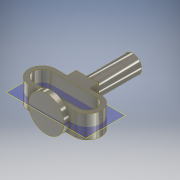
# Autodesk Inventor part: 부품1
Saved by Autodesk Inventor 2018 (Build 220112000, 112)
## iProperties
Created: 2019-05-21
Part Number: 부품1
Material: 은
Document SubType Name: Modeling
Designer: LeeYounSeo
Mass: 3715.59 g
Surface Area: 594.159 cm^2
Volume: 354.204 cm^3
Density: 10.49 g/cm^3
Appearance: 은
Author: LeeYounSeo
Autodesk Inventor part; units mm, degrees
ref_plane "YZ Plane" through (0, 0, 0) normal (1, 0, 0) x (0, 1, 0)
ref_plane "XZ Plane" through (0, 0, 0) normal (0, 1, 0) x (-1, 0, 0)
ref_plane "XY Plane" through (0, 0, 0) normal (0, 0, 1) x (1, 0, 0)
sketch "스케치1" plane through (0, 0, 0) normal (0, 0, 1) x (1, 0, 0)
  line L0 (-50, -20) -> (50, -20)
  line L1 (50, 20) -> (-50, 20)
  line L2 (-50, -20) -> (50, 20) construction
  line L3 (50, -20) -> (-50, 20) construction
  arc A0 (-50, 20) -> (-50, -20) centre (-50, 0) ccw
  arc A1 (50, -20) -> (50, 20) centre (50, 0) ccw
  arc A2 (50, -30) -> (50, 30) centre (50, 0) ccw
  line L4 (50, -30) -> (-50, -30)
  arc A3 (-50, 30) -> (-50, -30) centre (-50, 0) ccw
  line L5 (25, 30) -> (25, 50)
  line L6 (-25, 30) -> (-25, 50)
  line L7 (-50, 30) -> (-25, 30)
  line L8 (25, 30) -> (50, 30)
  line L9 (-25, 50) -> (25, 50)
  point P0 (0, 0)
  point P1 (0, 0)
  dimension "d13" = 20
  dimension "d14" = 10
  constraints: 20 end point, 8 point on circle, 4 centre point, 3 midpoint, 3 parallel, 2 horizontal, 2 tangent, 2 other
  measures "d13" radius of A1
  measures "d14" radial gap between concentric circles of A2 A1
extrude "돌출1" add sketch "스케치1" along normal blind 50
sketch "스케치2" plane through (-25, 50, 0) normal (0, 1, 0) x (1, 0, 0)
  point P0 (25, 0)
ref_plane "작업 평면1" through (0, 0, 25) normal (0, 0, -1) x (-1, 0, 0)
sketch "스케치3" plane through (-25, 50, 0) normal (0, 1, 0) x (1, 0, 0)
  circle A0 centre (25, -25.091) radius 20
  point P0 (25, 0)
  dimension "d17" = 40
  constraints: 1 centre point
  measures "d17" diameter of A0
extrude "돌출2" add sketch "스케치3" along normal blind 100
sketch "스케치4" plane through (0, 0, 25) normal (0, 0, -1) x (-1, 0, 0)
  line L0 (50, -30) -> (-50, -30) projected
  line L1 (0, -30) -> (39.4468, -30)
  line L2 (39.4468, -30) -> (39.4468, -41.4109)
  line L3 (39.4468, -41.4109) -> (0, -41.4109)
  line L4 (0, -41.4109) -> (0, -30)
  point P0 (0, 0)
  constraints: 8 end point, 2 parallel, 1 horizontal, 1 midpoint, 1 perpendicular
revolve "회전1" add sketch "스케치4" angle 360 about axis through (0, -41.4109, 25) along (0, 1, 0)
